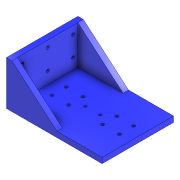
# Autodesk Inventor part: positioner_base
Saved by Autodesk Inventor 2022 (Build 260153000, 153)
## iProperties
Created: 2021-04-23
Part Number: positioner_base
Material: Generic
Document SubType Name: Modeling
Designer: nnico
Density: 1 g/cm^3
Appearance: Blue - Wall Paint - Glossy
Author: nnico
Autodesk Inventor part; units mm, degrees
ref_plane "YZ Plane" through (0, 0, 0) normal (1, 0, 0) x (0, 1, 0)
ref_plane "XZ Plane" through (0, 0, 0) normal (0, 1, 0) x (-1, 0, 0)
ref_plane "XY Plane" through (0, 0, 0) normal (0, 0, 1) x (1, 0, 0)
sketch "Sketch1" plane through (0, 0, 0) normal (0, 1, 0) x (-1, 0, 0)
  line L0 (20, -4.85) -> (-20, -4.85) construction
  line L1 (-20, -4.85) -> (-20, 4.85) construction
  line L2 (-20, 4.85) -> (20, 4.85) construction
  line L3 (20, 4.85) -> (20, -4.85) construction
  line L4 (0, -4.85) -> (0, 4.85) construction
  line L5 (20, 0) -> (-20, 0) construction
  circle A0 centre (13.5, 0) radius 2.25
  circle A1 centre (-13.5, 0) radius 2.25
  line L6 (67, -18) -> (25, -18) construction
  line L7 (25, -18) -> (25, 18) construction
  line L8 (25, 18) -> (67, 18) construction
  line L9 (67, 18) -> (67, -18) construction
  line L10 (46, -18) -> (46, 18) construction
  line L11 (67, 0) -> (25, 0) construction
  circle A2 centre (61.25, -13) radius 2.75
  circle A3 centre (30.75, -13) radius 2.75
  circle A4 centre (61.25, 13) radius 2.75
  circle A5 centre (30.75, 13) radius 2.75
  line L12 (-67, -18) -> (-25, -18) construction
  line L13 (-25, -18) -> (-25, 18) construction
  line L14 (-25, 18) -> (-67, 18) construction
  line L15 (-67, 18) -> (-67, -18) construction
  line L16 (-46, -18) -> (-46, 18) construction
  line L17 (-67, 0) -> (-25, 0) construction
  circle A6 centre (-61.25, -13) radius 2.75
  circle A7 centre (-30.75, -13) radius 2.75
  circle A8 centre (-61.25, 13) radius 2.75
  circle A9 centre (-30.75, 13) radius 2.75
  line L18 (82, -65) -> (-82, -65)
  line L19 (-82, -65) -> (-82, 65)
  line L20 (-82, 65) -> (82, 65)
  line L21 (82, 65) -> (82, -65)
  point P0 (0, 0)
  point P1 (0, 0)
  dimension "d0" = 40
  dimension "d1" = 9.7
  dimension "d2" = 4.5
  dimension "d3" = 27
  dimension "d4" = 42
  dimension "d6" = 36
  dimension "d7" = 5
  dimension "d8" = 5.5
  dimension "d9" = 30.5
  dimension "d10" = 26
  dimension "d12" = 15
  dimension "d16" = 130
  constraints: 44 end point, 16 symmetric about line, 10 centre point, 9 midpoint, 6 parallel, 3 horizontal, 3 perpendicular, 1 coincident, 1 collinear, 1 point on line, 10 other
  measures "d0" distance of L1.end L2.end
  measures "d1" distance of L0.end L1.end
  measures "d2" diameter of A0
  measures "d3" diameter of A0.centre L4
  measures "d4" distance of L7.end L8.end
  measures "d6" distance of L8.end L6.start
  measures "d7" distance between parallel lines of L3 L7
  measures "d8" diameter of A2
  measures "d9" diameter of A2.centre L10
  measures "d10" diameter of A2.centre L11
  measures "d12" distance from line of L19 L14.end
  measures "d16" distance of L18.end L19.end
extrude "Extrusion1" add sketch "Sketch1" along normal blind 10
sketch "Sketch5" plane through (-82, 0, -65) normal (-1, 0, 0) x (0, 0, 1)
  line L0 (0, 0) -> (130, 0) projected
  line L1 (130, 0) -> (130, 10) projected
  line L2 (0, 10) -> (130, 10) projected
  line L3 (0, 0) -> (0, 10) projected
  point P0 (65, 0)
extrude "Extrusion4" add sketch "Sketch5" along normal blind 10
sketch "Sketch6" plane through (0, 10, 0) normal (0, 1, 0) x (1, 0, 0)
  line L0 (-92, 65) -> (-92, -65) projected
  line L1 (82, -65) -> (-92, -65) projected
  line L2 (-92, 65) -> (-82, 65)
  line L3 (-82, 65) -> (-82, -65)
  line L4 (-82, -65) -> (-92, -65)
  line L5 (-92, -65) -> (-92, 65)
  point P0 (0, 0)
  dimension "d33" = 10
  constraints: 8 end point, 2 parallel, 1 horizontal, 1 perpendicular, 1 point on line
  measures "d33" distance of L3.end L4.end
extrude "Extrusion5" add sketch "Sketch6" along normal blind 80
sketch "Sketch7" plane through (-82, 10, 65) normal (1, 0, 0) x (0, 0, -1)
  line L0 (35, 10) -> (95, 10)
  line L1 (95, 10) -> (95, 70)
  line L2 (95, 70) -> (35, 70)
  line L3 (35, 70) -> (35, 10)
  line L4 (130, 80) -> (0, 80) construction
  line L5 (65, 80) -> (65, 0) construction
  line L6 (62.75, 0) -> (67.25, 0) construction
  line L7 (0, -10) -> (0, 80) construction
  line L8 (130, -10) -> (130, 80) construction
  line L9 (130, 40) -> (0, 40) construction
  point P0 (65, -10)
  dimension "d36" = 60
  dimension "d37" = 60
  dimension "d38" = 40
  constraints: 12 end point, 2 midpoint, 2 parallel, 2 perpendicular, 2 point on line, 1 horizontal, 2 other
  measures "d36" distance of L1.end L2.end
  measures "d37" distance of L0.end L1.end
  measures "d38" distance of L4.end L9.end
extrude "Extrusion6" add sketch "Sketch7" along normal blind 10
sketch "Sketch8" plane through (0, 90, 0) normal (0, 1, 0) x (1, 0, 0)
  line L0 (-92, 65) -> (-92, -65) projected
  line L1 (-92, -65) -> (-82, -65) projected
  line L2 (-82, -65) -> (-82, 65) projected
  line L3 (-82, 65) -> (-92, 65) projected
  point P0 (0, 0)
extrude "Extrusion7" cut sketch "Sketch8" against normal up to surface (10 mm away)
sketch "Sketch9" plane through (-72, 10, 65) normal (1, 0, 0) x (0, 0, -1)
  line L0 (95, 10) -> (95, 70) construction
  line L1 (95, 70) -> (35, 70) construction
  line L2 (35, 70) -> (35, 10) construction
  line L3 (35, 10) -> (95, 10) construction
  line L4 (35, 10) -> (35, 70) construction
  line L5 (35, 40) -> (95, 40) construction
  line L6 (95, 10) -> (95, 70) construction
  line L7 (35, 10) -> (95, 10) construction
  line L8 (65, 10) -> (65, 70) construction
  line L9 (95, 70) -> (35, 70) construction
  line L10 (41.45, 63.55) -> (88.55, 63.55) construction
  line L11 (88.55, 63.55) -> (88.55, 16.45) construction
  line L12 (88.55, 16.45) -> (41.45, 16.45) construction
  line L13 (41.45, 16.45) -> (41.45, 63.55) construction
  circle A0 centre (41.45, 63.55) radius 2.75
  circle A1 centre (41.45, 16.45) radius 2.75
  circle A2 centre (88.55, 16.45) radius 2.75
  circle A3 centre (88.55, 63.55) radius 2.75
  circle A4 centre (65, 40) radius 19.05
  point P0 (65, -10)
  dimension "d43" = 47.1
  dimension "d44" = 47.1
  dimension "d45" = 5.5
  dimension "d46" = 5.5
  dimension "d47" = 5.5
  dimension "d48" = 5.5
  dimension "d51" = 38.1
  constraints: 12 end point, 5 centre point, 5 midpoint, 4 coincident, 2 parallel, 1 horizontal, 1 perpendicular, 2 other
  measures "d43" distance of L11.end L12.end
  measures "d44" distance of L10.end L11.end
  measures "d45" diameter of A0
  measures "d46" diameter of A1
  measures "d47" diameter of A2
  measures "d48" diameter of A3
  measures "d51" diameter of A4
extrude "Extrusion8" cut sketch "Sketch9" against normal through all
sketch "Sketch10" plane through (-92, 0, -65) normal (-1, 0, 0) x (0, 0, 1)
  circle A0 centre (65, 50) radius 19.05 projected
  line L0 (65, 50) -> (0, 50) construction
  line L1 (0, 10) -> (0, 80) projected
  line L2 (65, 50) -> (130, 50) construction
  line L3 (130, 10) -> (130, 80) projected
  line L4 (5, 71.2) -> (33, 71.2) construction
  line L5 (33, 71.2) -> (33, 24.2) construction
  line L6 (33, 24.2) -> (5, 24.2) construction
  line L7 (5, 24.2) -> (5, 71.2) construction
  line L8 (5, 47.7) -> (33, 47.7) construction
  line L9 (65, 50) -> (65, 0) construction
  line L10 (19, 71.2) -> (19, 24.2) construction
  circle A1 centre (19, 65.7) radius 2.75
  circle A2 centre (19, 29.7) radius 2.75
  circle A3 centre (111, 65.7) radius 2.75
  circle A4 centre (111, 29.7) radius 2.75
  point P0 (180, 80)
  dimension "d52" = 28
  dimension "d53" = 47
  dimension "d54" = 2.3
  dimension "d55" = 46
  dimension "d56" = 5.5
  dimension "d57" = 36
  constraints: 18 end point, 4 centre point, 4 midpoint, 3 horizontal, 3 symmetric about line, 2 parallel, 2 point on line, 1 perpendicular, 1 vertical, 5 other
  measures "d52" distance of L5.end L6.end
  measures "d53" distance of L4.end L5.end
  measures "d54" distance from line of L0 L8.start
  measures "d55" distance from line of L9 L10.end
  measures "d56" diameter of A1
  measures "d57" diameter of A1.centre L8
extrude "Extrusion9" cut sketch "Sketch10" against normal through all contours A1 | A2 | A3 | A4
sketch "Sketch12" plane through (0, 10, 0) normal (0, 1, 0) x (1, 0, 0)
  line L0 (82, 65) -> (-82, 65) projected
  line L1 (-82, 65) -> (0, 65)
  line L2 (0, 65) -> (0, 55)
  line L3 (0, 55) -> (-82, 55)
  line L4 (-82, 55) -> (-82, 65)
  line L5 (82, -65) -> (82, 65) construction
  line L6 (82, 0) -> (-92, 0) construction
  line L7 (-92, 65) -> (-92, -65) construction
  line L8 (-82, -65) -> (0, -65)
  line L9 (0, -65) -> (0, -55)
  line L10 (0, -55) -> (-82, -55)
  line L11 (-82, -55) -> (-82, -65)
  point P0 (0, 0)
  dimension "d70" = 82
  dimension "d71" = 10
  constraints: 18 end point, 4 symmetric about line, 2 midpoint, 2 parallel, 1 horizontal, 1 perpendicular
  measures "d70" distance of L2.end L3.end
  measures "d71" distance of L1.end L2.end
extrude "Extrusion11" add sketch "Sketch12" along normal up to surface (70 mm away)
chamfer "Chamfer3" distance 70 distance2 82 1 edges at (0, 80, -60) measured on face at (0, 33.3333, -58.3333)
chamfer "Chamfer4" distance 70 distance2 82 1 edges at (0, 80, 60) measured on face at (0, 33.3333, 61.6667)
sketch "Sketch13" plane through (-72, 10, 65) normal (1, 0, 0) x (0, 0, -1)
  line L0 (95, 10) -> (35, 10) projected
  line L1 (95, 10) -> (95, 70) projected
  line L2 (35, 10) -> (95, 10)
  line L3 (95, 10) -> (95, 70)
  line L4 (95, 70) -> (35, 70)
  line L5 (35, 70) -> (35, 10)
  point P0 (65, -10)
  constraints: 8 end point, 2 parallel, 1 horizontal, 1 perpendicular
extrude "Extrusion12" add sketch "Sketch13" against normal blind 20
sketch "Sketch14" plane through (-72, 10, 65) normal (1, 0, 0) x (0, 0, -1)
  line L0 (95, 10) -> (95, 70) projected
  line L1 (95, 70) -> (35, 70) projected
  line L2 (35, 70) -> (35, 10) projected
  line L3 (35, 10) -> (95, 10) projected
  point P0 (65, -10)
extrude "Extrusion13" cut sketch "Sketch14" against normal blind 10
sketch "Sketch15" plane through (-92, 0, -65) normal (-1, 0, 0) x (0, 0, 1)
  circle A0 centre (19, 29.7) radius 2.75 construction
  circle A1 centre (19, 65.7) radius 2.75 construction
  line L0 (19, 29.7) -> (19, 65.7) construction
  circle A2 centre (111, 29.7) radius 2.75 construction
  circle A3 centre (111, 65.7) radius 2.75 construction
  line L1 (111, 29.7) -> (111, 65.7) construction
  line L2 (19, 47.7) -> (111, 47.7) construction
  line L3 (51.5, 74) -> (78.5, 74) construction
  line L4 (78.5, 74) -> (78.5, 26) construction
  line L5 (78.5, 26) -> (51.5, 26) construction
  line L6 (51.5, 26) -> (51.5, 74) construction
  line L7 (51.5, 50) -> (78.5, 50) construction
  line L8 (130, 80) -> (0, 80) construction
  line L9 (65, 80) -> (65, 0) construction
  line L10 (65, 74) -> (65, 26) construction
  circle A4 centre (65, 68.3) radius 2.75
  circle A5 centre (65, 31.7) radius 2.75
  dimension "d84" = 27
  dimension "d85" = 48
  dimension "d86" = 2.3
  dimension "d87" = 5.5
  dimension "d88" = 36.6
  constraints: 20 end point, 7 midpoint, 3 vertical, 2 centre point, 2 parallel, 1 collinear, 1 horizontal, 1 perpendicular, 1 point on line, 1 symmetric about line, 1 other
  measures "d84" distance of L4.end L5.end
  measures "d85" distance of L3.end L4.end
  measures "d86" distance between parallel lines of L2 L7
  measures "d87" diameter of A4
  measures "d88" diameter of A4.centre L7
extrude "Extrusion14" cut sketch "Sketch15" against normal blind 10
body "Solid1"
